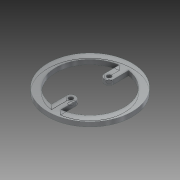
# Autodesk Inventor part: TreeHolder
Saved by Autodesk Inventor 2014 (Build 180170000, 170)
## iProperties
Created: 2013-12-17
Part Number: TreeHolder
Material: Generic
Document SubType Name: Modeling
Designer: blacki
Density: 1 g/cm^3
Appearance: Clear Reflective
Author: blacki
Autodesk Inventor part; units mm, degrees
ref_plane "YZ Plane" through (0, 0, 0) normal (1, 0, 0) x (0, 1, 0)
ref_plane "XZ Plane" through (0, 0, 0) normal (0, 1, 0) x (-1, 0, 0)
ref_plane "XY Plane" through (0, 0, 0) normal (0, 0, 1) x (1, 0, 0)
sketch "Sketch1" plane through (0, 0, 0) normal (0, 0, 1) x (1, 0, 0)
  circle A0 centre (0, 0) radius 27.5
  dimension "d0" = 55
  constraints: 1 centre point, 1 coincident
  measures "d0" diameter of A0
extrude "Extrusion1" add sketch "Sketch1" along normal blind 3
sketch "Sketch2" plane through (0, 0, 3) normal (0, 0, 1) x (1, 0, 0)
  circle A0 centre (0, 0) radius 27.5 projected
  circle A1 centre (0, 0) radius 22.5
  dimension "d3" = 45
  constraints: 1 centre point
  measures "d3" diameter of A1
extrude "Extrusion2" cut sketch "Sketch2" against normal up to next contours A1
sketch "Sketch4" plane through (0, 0, 3) normal (0, 0, 1) x (1, 0, 0)
  circle A0 centre (0, 0) radius 22.5 projected
  line L0 (0, 12.5) -> (0, 22.5) construction
  line L1 (-3, 12.5) -> (-3, 22.5)
  line L2 (3, 22.5) -> (3, 12.5)
  arc A1 (-3, 12.5) -> (3, 12.5) centre (0, 12.5) ccw
  arc A2 (3, 22.5) -> (-3, 22.5) centre (0, 22.5) ccw
  point P0 (0, 17.5)
  dimension "d10" = 10
  dimension "d11" = 6
  constraints: 8 end point, 4 point on circle, 4 tangent, 2 centre point, 1 midpoint, 1 parallel, 1 vertical, 1 vertical alignment, 1 other
  measures "d10" distance of L0.start L0.end
  measures "d11" distance between parallel lines of L2 L1
extrude "Extrusion4" add sketch "Sketch4" against normal up to surface (3 mm away) contours L2 A1 L1 A0 | A0 L1 A2 L2 picked at (-0.3342, 15.8259)
hole "Hole1" at (0, 12.5, 3) direction (0, 0, -1) diameter 3 end through all
mirror "Mirror1" about plane through (0, 0, 0) normal (0, 1, 0) of "Extrusion4", "Hole1"
body "Solid1"
